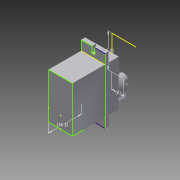
# Autodesk Inventor part: HD-1900A_Servo
Saved by Autodesk Inventor 2015 (Build 190159000, 159)
## iProperties
Created: 2014-10-28
Part Number: HD-1900A_Servo
Material: ABS Plastic
Document SubType Name: Modeling
Designer: s4201025
Density: 1.06 g/cm^3
Appearance: Smooth - White
Author: s4201025
Autodesk Inventor part; units mm, degrees
ref_plane "YZ Plane" through (0, 0, 0) normal (1, 0, 0) x (0, 1, 0)
ref_plane "XZ Plane" through (0, 0, 0) normal (0, 1, 0) x (-1, 0, 0)
ref_plane "XY Plane" through (0, 0, 0) normal (0, 0, 1) x (1, 0, 0)
sketch "Sketch1" plane through (0, 0, 0) normal (0, 1, 0) x (-1, 0, 0)
  line L0 (-6, -6) -> (6, -6)
  line L1 (6, -6) -> (6, 16.9)
  line L2 (6, 16.9) -> (-6, 16.9)
  line L3 (-6, 16.9) -> (-6, -6)
  point P0 (0, 0)
  dimension "d0" = 12
  dimension "d1" = 22.9
  constraints: 8 end point, 2 parallel, 1 horizontal, 1 perpendicular
  measures "d0" distance of L2.end L1.end
  measures "d1" distance of L1.end L0.end
extrude "Extrusion1" add sketch "Sketch1" along normal blind 16.3
sketch "Sketch2" plane through (0, 16.3, 0) normal (0, 1, 0) x (1, 0, 0)
  line L0 (6, 10.8) -> (6, -21.7)
  line L1 (-6, -21.7) -> (-6, 10.8)
  line L2 (6, 8.55) -> (6, -19.45)
  line L3 (-6, -19.45) -> (-6, 8.55)
  arc A0 (-0.5, 9.416) -> (0.5, 9.416) centre (0, 8.55) ccw
  line L4 (0.5, 10.8) -> (0.5, 9.416)
  line L5 (-0.5, 10.8) -> (-0.5, 9.416)
  line L6 (-6, 10.8) -> (-0.5, 10.8)
  line L7 (0.5, 10.8) -> (6, 10.8)
  arc A1 (0.5, -20.316) -> (-0.5, -20.316) centre (0, -19.45) ccw
  line L8 (-0.5, -21.7) -> (-0.5, -20.316)
  line L9 (0.5, -21.7) -> (0.5, -20.316)
  line L10 (6, -21.7) -> (0.5, -21.7)
  line L11 (-0.5, -21.7) -> (-6, -21.7)
  line L12 (-6, -16.9) -> (6, -16.9) projected
  line L13 (6, 6) -> (-6, 6) projected
  point P0 (0, 0)
  dimension "d5" = 32.5
  dimension "d12" = 28
  dimension "d28" = 27.7
  dimension "d29" = 22.9
  dimension "d32" = 2.55
  dimension "d33" = 4.8
  dimension "d34" = 1
  dimension "d35" = 12
  constraints: 24 end point, 6 parallel, 4 point on circle, 2 centre point, 2 horizontal, 2 perpendicular
  measures "d5" distance of L0.start L0.end
  measures "d12" distance of L2.start L2.end
  measures "d28" distance between parallel lines of L12 L7
  measures "d29" distance between parallel lines of L12 L13
  measures "d32" distance from line of L13 A0.centre
  measures "d33" distance between parallel lines of L7 L13
  measures "d34" radius of A0
  measures "d35" distance between parallel lines of L1 L0
extrude "Extrusion2" add sketch "Sketch2" along normal blind 2
sketch "Sketch3" plane through (0, 18.3, 0) normal (0, 1, 0) x (1, 0, 0)
  line L0 (-6, 6) -> (6, 6)
  line L1 (6, 6) -> (6, -16.9)
  line L2 (6, -16.9) -> (-6, -16.9)
  line L3 (-6, -16.9) -> (-6, 6)
  point P0 (0, 0)
  dimension "d9" = 22.9
  constraints: 8 end point, 2 parallel, 1 horizontal, 1 perpendicular
  measures "d9" distance of L0.end L1.end
extrude "Extrusion3" add sketch "Sketch3" along normal blind 4.9
sketch "Sketch4" plane through (0, 23.2, 0) normal (0, 1, 0) x (1, 0, 0)
  arc A0 (2.3077, -5.5385) -> (-2.3077, -5.5385) centre (0, 0) ccw
  arc A1 (-2.3077, -5.5385) -> (2.3077, -5.5385) centre (0, -6.5) ccw
  constraints: 4 point on circle, 2 centre point
extrude "Extrusion4" add sketch "Sketch4" along normal blind 4.1
sketch "Sketch5" plane through (0, 27.3, 0) normal (0, 1, 0) x (1, 0, 0)
  circle A0 centre (0, 0) radius 2.5
  dimension "d18" = 5
  constraints: 1 centre point
  measures "d18" diameter of A0
extrude "Extrusion5" add sketch "Sketch5" along normal blind 4.4
sketch "Sketch6" plane through (6, 0, -6) normal (0, 0, -1) x (-1, 0, 0)
  line L0 (0, 0) -> (0, 5.5)
  line L1 (0, 5.5) -> (12, 5.5)
  line L2 (6, 4) -> (8.125, 4)
  line L3 (3.875, 4) -> (8.125, 4)
  line L4 (8.125, 4) -> (8.125, 5.5)
  line L5 (8.125, 5.5) -> (3.875, 5.5)
  line L6 (3.875, 5.5) -> (3.875, 4)
  point P0 (6, 0)
  dimension "d22" = 5.5
  dimension "d23" = 4.25
  constraints: 14 end point, 2 parallel, 1 horizontal, 1 midpoint, 1 perpendicular
  measures "d22" distance of L0.start L0.end
  measures "d23" distance of L5.end L4.end
extrude "Extrusion6" add sketch "Sketch6" along normal blind 1
sketch "Sketch7" plane through (0, 31.7, 0) normal (0, 1, 0) x (1, 0, 0)
  line L0 (-6, -16.9) -> (6, -16.9) projected
  line L1 (-6, 0) -> (-6, -16.9) projected
  point P0 (0, 0)
  dimension "d26" = 16.9
  dimension "d27" = 6
  measures "d26" distance from line of L0 point (0, 0)
  measures "d27" distance from line of L1 point (0, 0)
sketch "Sketch8" plane through (-6, 0, -6) normal (-1, 0, 0) x (0, 0, 1)
  line L0 (0, 0) -> (22.9, 0) projected
  line L1 (-4.8, 16.3) -> (0, 16.3) projected
  point P0 (6, 0)
  dimension "d30" = 16.3
  measures "d30" distance between parallel lines of L0 L1
body "Solid1"
